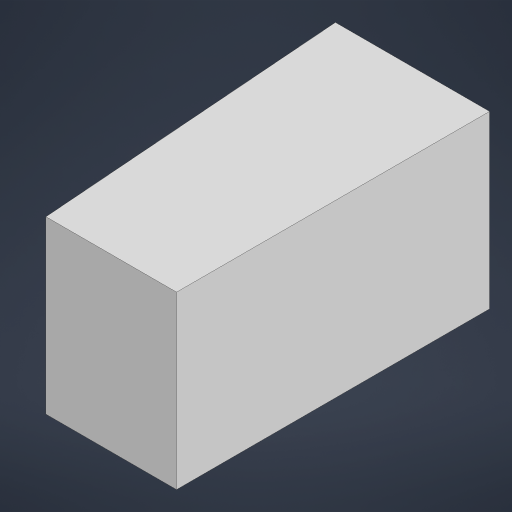
# Autodesk Inventor part: Part1
Saved by Autodesk Inventor 2023 (Build 270158000, 158)
## iProperties
Created: 2023-08-21
Part Number: Part1
Material: Generic
Document SubType Name: Modeling
Designer: Zain Ali
Density: 1 g/cm^3
Appearance: Default
Author: Zain Ali
Autodesk Inventor part; units mm, degrees
ref_plane "YZ Plane" through (0, 0, 0) normal (1, 0, 0) x (0, 1, 0)
ref_plane "XZ Plane" through (0, 0, 0) normal (0, 1, 0) x (-1, 0, 0)
ref_plane "XY Plane" through (0, 0, 0) normal (0, 0, 1) x (1, 0, 0)
sketch "Sketch1" plane through (0, 0, 0) normal (0, 1, 0) x (-1, 0, 0)
  line L0 (9.7, 19.4) -> (-9.7, 19.4)
  line L1 (-9.7, 19.4) -> (-9.7, -27.1)
  line L2 (-9.7, -27.1) -> (13.2, -27.1)
  line L3 (9.7, 19.4) -> (13.2, -27.1)
  point P0 (0, 0)
  dimension "d6" = 19.4
  dimension "d7" = 46.5
  dimension "d8" = 22.9
  constraints: 8 end point, 1 horizontal, 1 parallel, 1 perpendicular
  measures "d6" distance of L0.start L0.end
  measures "d7" distance of L0.end L1.end
  measures "d8" distance of L1.end L2.end
extrude "Extrusion1" add sketch "Sketch1" along normal blind 25.4
body "Solid1"
